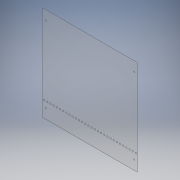
# Autodesk Inventor part: Lateral Acrilico
Saved by Autodesk Inventor 2018 (Build 220112000, 112)
## iProperties
Created: 2018-07-06
Part Number: Lateral Acrilico
Material: PMMA plástico
Document SubType Name: Chapa de metal
Designer: Regner
Density: 1.188 g/cm^3
Sheet Metal Rule: Padrão_mm
Appearance: Policarbonato - Transparente
Author: Regner
Autodesk Inventor part; units mm, degrees
ref_plane "YZ Plane" through (0, 0, 0) normal (1, 0, 0) x (0, 1, 0)
ref_plane "XZ Plane" through (0, 0, 0) normal (0, 1, 0) x (-1, 0, 0)
ref_plane "XY Plane" through (0, 0, 0) normal (0, 0, 1) x (1, 0, 0)
sketch "Esboço2" plane through (0, 0, 0) normal (0, 1, 0) x (-1, 0, 0)
  line L0 (-150, 150) -> (150, 150)
  line L1 (150, 150) -> (150, -150)
  line L2 (150, -150) -> (-150, -150)
  line L3 (-150, -150) -> (-150, 150)
  line L4 (-150, 150) -> (150, -150) construction
  line L5 (150, 150) -> (-150, -150) construction
  point P0 (0, 0)
  dimension "d2" = 300
  dimension "d3" = 300
  measures "d2" distance of L1.end L2.end
  measures "d3" distance of L0.end L1.end
extrude "Placa1" add sketch "Esboço2" along normal blind 0.5
sketch "Esboço3" plane through (0, 0.5, 0) normal (0, 1, 0) x (1, 0, 0)
  line L0 (150, -150) -> (-150, -150) projected
  line L1 (-150, -150) -> (-150, 150) projected
  point P0 (0, 0)
  point P1 (-140, -120)
  point P2 (140, -120)
  point P3 (-140, 120)
  point P4 (140, 120)
  dimension "d5" = 120
  dimension "d6" = 140
  dimension "d9" = 280
  dimension "d12" = 240
  constraints: 1 horizontal, 1 vertical, 3 other
  measures "d5" vertical distance of point (0, 0) point (-140, -120)
  measures "d6" horizontal distance of point (0, 0) point (-140, -120)
  measures "d9" distance of point (-140, -120) point (140, -120)
  measures "d12" distance of point (-140, -120) point (-140, 120)
hole "Furo1" at (-140, 0.5, 120) at (140, 0.5, 120) at (-140, 0.5, -120) at (140, 0.5, -120) direction (0, -1, 0) diameter 4 end through all
sketch "Esboço4" plane through (0, 0, 0) normal (0, -1, 0) x (1, 0, 0)
  circle A0 centre (-145, -100) radius 2.5
  line L0 (-150, 150) -> (-150, -150) projected
  line L1 (-150, -150) -> (150, -150) projected
  point P0 (0, 0)
  dimension "d22" = 5
  dimension "d23" = 5
  dimension "d24" = 50
  constraints: 1 centre point
  measures "d22" diameter of A0
  measures "d23" distance from line of L0 A0.centre
  measures "d24" distance from line of L1 A0.centre
extrude "Extrusão1" cut sketch "Esboço4" against normal up to surface (0.5 mm away)
pattern_linear "Padrão retangular1" count 30 spacing 10 along (1, 0, 0) of "Extrusão1"
equation "\"d9\" = 2 * d6"
equation "\"d12\" = 2 * d5"
equation "\"d20\" = Espessura"
equation "\"d4\" = Espessura"
equation "\"Raio_vergadura\" = Espessura"
equation "\"Largura_alívio_de_vergadura\" = Espessura"
equation "\"Profundidade_alívio_de_vergadura\" = 0.5 * Espessura"
equation "\"Tamanho_alívio_de_dobra\" = 4 * Espessura"
equation "\"Remanescente_mínimo\" = 2 * Espessura"
equation "\"Raiodetransição\" = Raio_vergadura"
equation "\"Tamanho_de_raio_de_Jacobi\" = Raio_vergadura"
equation "\"TamanhoFolga\" = Espessura"
equation "\"Espessura\" = 0.5"
